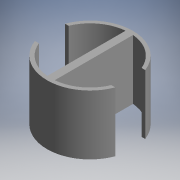
# Autodesk Inventor part: Electronics_Bay_2Inch
Saved by Autodesk Inventor 2018 (Build 220112000, 112)
## iProperties
Part Number: Electronics_Bay_2Inch
Material: Generic
Document SubType Name: Modeling
Designer: Intel
Appearance: Generic
Author: Intel
Autodesk Inventor part; units mm, degrees
ref_plane "YZ Plane" through (0, 0, 0) normal (1, 0, 0) x (0, 1, 0)
ref_plane "XZ Plane" through (0, 0, 0) normal (0, 1, 0) x (-1, 0, 0)
ref_plane "XY Plane" through (0, 0, 0) normal (0, 0, 1) x (1, 0, 0)
sketch "Sketch1" plane through (0, 0, 0) normal (0, 1, 0) x (-1, 0, 0)
  line L0 (-47.0591, 0) -> (40.0927, 0) construction
  line L1 (0, 56.4222) -> (0, -48.8199) construction
  arc A0 (34.2324, 12.6999) -> (-34.2324, 12.6999) centre (0, 0) ccw
  arc A1 (-34.1876, -12.8208) -> (34.1876, -12.8208) centre (0, 0) ccw
  line L2 (-34.2324, 12.6999) -> (-30.8234, 12.6999)
  line L3 (30.8234, 12.6999) -> (34.2324, 12.6999)
  line L4 (34.1876, -12.8208) -> (31.1169, -12.8208)
  line L5 (-31.1169, -12.8208) -> (-34.1876, -12.8208)
  line L6 (-3.175, 33.1857) -> (-3.175, -33.5045)
  arc A2 (30.8234, 12.6999) -> (3.175, 33.1857) centre (0, 0) ccw
  arc A3 (-3.175, 33.1857) -> (-30.8234, 12.6999) centre (0, 0) ccw
  line L7 (3.175, -33.5045) -> (3.175, 33.1857)
  arc A4 (-31.1169, -12.8208) -> (-3.175, -33.5045) centre (0, 0) ccw
  arc A5 (3.175, -33.5045) -> (31.1169, -12.8208) centre (0, 0) ccw
  dimension "d16" = 3.175
  dimension "d17" = 3.175
  constraints: 16 end point, 12 point on circle, 6 centre point, 5 parallel, 4 horizontal, 2 vertical, 1 coincident, 2 other
  measures "d16" distance between parallel lines of L7 L1
  measures "d17" distance between parallel lines of L6 L1
extrude "Extrusion1" add sketch "Sketch1" along normal blind 50.8
equation "\"d13\" = 0.5 * d11"
equation "\"d11\" = 25.4"
body "Solid1"
